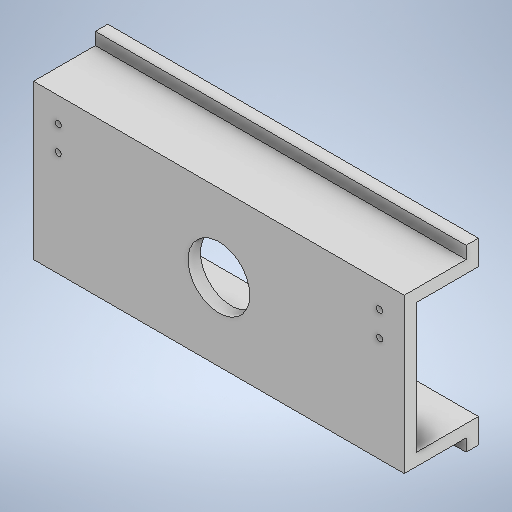
# Autodesk Inventor part: WheelCorver
Saved by Autodesk Inventor 2025.3 (Build 293356000, 356)
## iProperties
Created: 2025-04-27
Part Number: WheelCorver
Material: 일반
Document SubType Name: Modeling
Designer: SEON
Density: 1 g/cm^3
Appearance: 기본값
Author: SEON
Autodesk Inventor part; units mm, degrees
ref_plane "YZ Plane" through (0, 0, 0) normal (1, 0, 0) x (0, 1, 0)
ref_plane "XZ Plane" through (0, 0, 0) normal (0, 1, 0) x (-1, 0, 0)
ref_plane "XY Plane" through (0, 0, 0) normal (0, 0, 1) x (1, 0, 0)
sketch "스케치1" plane through (0, 0, 0) normal (0, 0, 1) x (1, 0, 0)
  line L0 (0, 0) -> (300, 0)
  line L1 (300, 0) -> (300, -145)
  line L2 (300, -145) -> (0, -145)
  line L3 (0, -145) -> (0, 0)
  line L4 (0, -20) -> (300, -20)
  line L5 (0, -125) -> (300, -125)
  line L6 (300, -135) -> (0, -135)
  line L7 (300, -10) -> (0, -10)
  dimension "d0" = 300
  dimension "d1" = 145
  dimension "d2" = 20
  dimension "d3" = 20
  dimension "d8" = 10
  dimension "d9" = 10
  constraints: 16 end point, 8 point on line, 5 perpendicular, 2 parallel, 1 horizontal
  measures "d0" distance of L0.start L0.end
  measures "d1" distance of L2.end L0.start
  measures "d2" distance between parallel lines of L2 L5
  measures "d3" distance between parallel lines of L0 L4
  measures "d8" distance between parallel lines of L2 L6
  measures "d9" distance between parallel lines of L7 L4
extrude "돌출1" add sketch "스케치1" along normal blind 10 contours L7 L1 L4 L3 | L4 L1 L5 L3 | L5 L1 L6 L3
extrude "돌출2" add sketch "스케치1" against normal blind 50 contours L0 L1 L7 L3 | L7 L1 L4 L3 | L5 L1 L6 L3 | L6 L1 L2 L3
extrude "돌출3" cut sketch "스케치1" against normal blind 40 contours L0 L1 L7 L3 | L6 L1 L2 L3
sketch "스케치2" plane through (0, 0, 10) normal (0, 0, 1) x (1, 0, 0)
  circle A0 centre (20, -30) radius 2.5
  circle A1 centre (280, -30) radius 2.5
  line L0 (300, -135) -> (300, -10) projected
  line L1 (0, -10) -> (0, -135) projected
  line L2 (0, 0) -> (300, 0) projected
  circle A2 centre (20, -50) radius 2.5
  circle A3 centre (280, -50) radius 2.5
  circle A4 centre (150, -72.5) radius 25
  point P0 (0, -72.5)
  point P1 (0, -72.5)
  point P2 (150, 0)
  dimension "d14" = 20
  dimension "d15" = 20
  dimension "d16" = 5
  dimension "d17" = 30
  dimension "d18" = 5
  dimension "d19" = 20
  dimension "d20" = 50
  constraints: 5 centre point, 3 horizontal alignment, 3 midpoint, 3 vertical alignment, 2 equal radius
  measures "d14" distance from line of L0 A1.centre
  measures "d15" horizontal distance of point (0, -72.5) A0.centre
  measures "d16" diameter of A0
  measures "d17" distance from line of L2 A0.centre
  measures "d18" diameter of A2
  measures "d19" distance of A1.centre A3.centre
  measures "d20" diameter of A4
extrude "돌출4" cut sketch "스케치2" against normal through all
equation "\"d8\" = 0.5 * d2"
equation "\"d9\" = d8"
